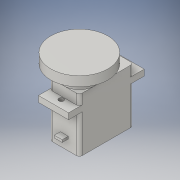
# Autodesk Inventor part: servo (2)
Saved by Autodesk Inventor 2016 (Build 200138000, 138)
## iProperties
Created: 2015-11-20
Part Number: servo (2)
Material: Generic
Document SubType Name: Modeling
Designer: Wilsonjame
Density: 1 g/cm^3
Appearance: White
Mass: 7.59956 g
Surface Area: 27.3499 cm^2
Volume: 7.59956 cm^3
Author: Wilsonjame
Autodesk Inventor part; units mm, degrees
ref_plane "YZ Plane" through (0, 0, 0) normal (1, 0, 0) x (0, 1, 0)
ref_plane "XZ Plane" through (0, 0, 0) normal (0, 1, 0) x (-1, 0, 0)
sketch "Sketch1" plane through (0, 0, 0) normal (0, 1, 0) x (-1, 0, 0)
  line L0 (1.27, 0) -> (11.43, 0)
  line L1 (12.7, -1.27) -> (12.7, -21.59)
  line L2 (11.43, -22.86) -> (1.27, -22.86)
  line L3 (0, -21.59) -> (0, -1.27)
  arc A0 (12.7, -1.27) -> (11.43, 0) centre (11.43, -1.27) ccw
  arc A1 (1.27, 0) -> (0, -1.27) centre (1.27, -1.27) ccw
  arc A2 (0, -21.59) -> (1.27, -22.86) centre (1.27, -21.59) ccw
  arc A3 (11.43, -22.86) -> (12.7, -21.59) centre (11.43, -21.59) ccw
  point P0 (0, 0)
  point P1 (12.7, -22.86)
  point P2 (12.7, 0)
  point P3 (0, -22.86)
  dimension "d0" = 12.7
  dimension "d1" = 22.86
  dimension "d2" = 1.27
  constraints: 8 end point, 8 point on circle, 8 point on line, 8 tangent, 4 centre point, 3 equal radius, 2 parallel, 1 horizontal, 1 perpendicular
  measures "d0" distance of point (12.7, -22.86) point (0, -22.86)
  measures "d1" distance of point (12.7, 0) point (12.7, -22.86)
  measures "d2" radius of A0
extrude "Extrusion1" add sketch "Sketch1" along normal blind 22.86
sketch "Sketch2" plane through (0, 22.86, 0) normal (0, 1, 0) x (1, 0, 0)
  line L0 (-12.7, 21.59) -> (-12.7, 1.27) projected
  line L1 (-11.43, 0) -> (-1.27, 0) projected
  line L2 (0, 1.27) -> (0, 21.59) projected
  circle A0 centre (-6.35, 6.35) radius 6.35
  point P0 (0, 0)
  constraints: 3 tangent, 1 centre point
extrude "Extrusion2" add sketch "Sketch2" along normal blind 5.08
sketch "Sketch3" plane through (-6.35, 27.94, -6.35) normal (0, 1, 0) x (1, 0, 0)
  circle A0 centre (0, 0) radius 12.065
  point P0 (6.35, -6.35)
  dimension "d9" = 24.13
  constraints: 1 centre point
  measures "d9" diameter of A0
extrude "Extrusion3" add sketch "Sketch3" along normal blind 4.064
ref_plane "Work Plane1" through (0, 18.542, 0) normal (0, 1, 0) x (1, 0, 0)
sketch "Sketch5" plane through (0, 18.542, 0) normal (0, 1, 0) x (1, 0, 0)
  line L0 (-12.7, 27.432) -> (0, 27.432)
  line L1 (-12.7, 21.59) -> (-12.7, 1.27) projected
  line L2 (0, 1.27) -> (0, 21.59) projected
  circle A0 centre (-6.35, 24.13) radius 1.016
  line L3 (0, 11.43) -> (-12.7, 11.43) construction
  line L4 (-12.7, -4.572) -> (0, -4.572)
  circle A1 centre (-6.35, -1.27) radius 1.016
  line L5 (-12.7, -4.572) -> (-12.7, 27.432)
  line L6 (0, 27.432) -> (0, -4.572)
  point P0 (0, 0)
  dimension "d13" = 16.002
  dimension "d14" = 2.032
  dimension "d15" = 25.4
  constraints: 10 end point, 3 symmetric about line, 2 centre point, 2 collinear, 2 midpoint, 1 horizontal, 1 perpendicular, 1 other
  measures "d13" distance from line of L0 L3.end
  measures "d14" diameter of A0
  measures "d15" distance of A0.centre A1.centre
extrude "Extrusion4" add sketch "Sketch5" against normal blind 2.54
sketch "Sketch6" plane through (-11.43, 0, 0) normal (0, 0, 1) x (1, 0, 0)
  line L0 (3.429, 5.334) -> (6.731, 5.334)
  line L1 (6.731, 5.334) -> (6.731, 4.318)
  line L2 (6.731, 4.318) -> (3.429, 4.318)
  line L3 (3.429, 4.318) -> (3.429, 5.334)
  line L4 (0, 0) -> (10.16, 0) projected
  point P0 (11.43, 0)
  point P1 (5.08, 0)
  point P2 (5.08, 4.318)
  dimension "d18" = 3.302
  dimension "d19" = 1.016
  dimension "d20" = 4.318
  constraints: 8 end point, 2 midpoint, 2 parallel, 1 horizontal, 1 perpendicular, 1 vertical alignment
  measures "d18" distance of L1.end L2.end
  measures "d19" distance of L0.end L1.end
  measures "d20" distance between parallel lines of L4 L2
extrude "Extrusion5" add sketch "Sketch6" along normal blind 2.54
body "Solid1"
